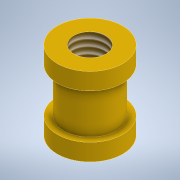
# Autodesk Inventor part: M3_tread_insert
Saved by Autodesk Inventor 2021 (Build 250183000, 183)
## iProperties
Created: 2022-06-30
Part Number: M3_tread_insert
Material: Generic
Document SubType Name: Modeling
Designer: lenna
Density: 1 g/cm^3
Appearance: Gold
Author: lenna
Autodesk Inventor part; units mm, degrees
ref_plane "YZ Plane" through (0, 0, 0) normal (1, 0, 0) x (0, 1, 0)
ref_plane "XZ Plane" through (0, 0, 0) normal (0, 1, 0) x (-1, 0, 0)
ref_plane "XY Plane" through (0, 0, 0) normal (0, 0, 1) x (1, 0, 0)
sketch "Sketch1" plane through (0, 0, 0) normal (0, 0, 1) x (1, 0, 0)
  line L0 (0, 3) -> (0, -3)
  line L1 (0, -3) -> (2.5, -3)
  line L2 (2.5, -3) -> (2.5, -1.7)
  line L3 (2.5, -1.7) -> (2, -1.7)
  line L4 (2, -1.7) -> (2, 1.7)
  line L5 (2, 1.7) -> (2.5, 1.7)
  line L6 (2.5, 1.7) -> (2.5, 3)
  line L7 (2.5, 3) -> (0, 3)
  point P0 (0, 0)
  dimension "d0" = 6
  dimension "d1" = 3
  dimension "d2" = 4
  dimension "d3" = 5
  dimension "d4" = 1.3
  dimension "d5" = 1.3
  constraints: 16 end point, 6 perpendicular, 2 point on line, 1 midpoint, 1 vertical
  measures "d0" distance between parallel lines of L1 L7
  measures "d1" distance from line of point (0, 0) L7
  measures "d2" diameter of L4 L0
  measures "d3" diameter of L6 L0
  measures "d4" distance between parallel lines of L7 L5
  measures "d5" distance between parallel lines of L1 L3
revolve "Revolution1" add sketch "Sketch1" angle 360 about axis through (0, 3, 0) along (0, -1, 0)
sketch "Sketch2" plane through (0, 3, 0) normal (0, 1, 0) x (1, 0, 0)
  circle A0 centre (0, 0) radius 2 projected
  point P0 (0, 0)
  constraints: 1 coincident
hole "Hole1" at (0, 3, 0) direction (0, -1, 0) diameter 2.459 depth 6 thread size "M3x0.5" class "6H" standard "ANSI Metric M Profile"
equation "\"d1\" = 0.5 * d0"
equation "\"d5\" = d4"
body "Solid1"
